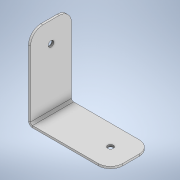
# Autodesk Inventor part: clamp
Saved by Autodesk Inventor 2021 (Build 250183000, 183)
## iProperties
Created: 2021-07-10
Part Number: clamp
Material: Generic
Document SubType Name: Sheet Metal
Designer: TARUN
Density: 1 g/cm^3
Sheet Metal Rule: Default_mm
Appearance: Default
Author: TARUN
Autodesk Inventor part; units mm, degrees
ref_plane "YZ Plane" through (0, 0, 0) normal (1, 0, 0) x (0, 1, 0)
ref_plane "XZ Plane" through (0, 0, 0) normal (0, 1, 0) x (-1, 0, 0)
ref_plane "XY Plane" through (0, 0, 0) normal (0, 0, 1) x (1, 0, 0)
sketch "Sketch1" plane through (0, 0, 0) normal (0, 1, 0) x (-1, 0, 0)
  line L0 (0, 5) -> (-20, 5)
  line L1 (-20, 5) -> (-20, -5)
  line L2 (-20, -5) -> (0, -5)
  line L3 (0, -5) -> (0, 5)
  point P0 (0, 0)
  dimension "d0" = 20
  dimension "d1" = 10
  measures "d0" distance of L0.start L0.end
  measures "d1" distance of L0.end L1.end
extrude "Plate1" add sketch "Sketch1" along normal blind 0.5
fillet "Corner Round1" radius 3 2 edges at (20, 0.25, 5) (20, 0.25, -5)
sketch "Sketch3" plane through (0, 0.5, 0) normal (0, 1, 0) x (1, 0, 0)
  line L0 (0, 5) -> (17, 5) projected
  line L1 (20, 2) -> (20, -2) projected
  point P0 (0, 0)
  point P1 (15, 0)
  point P2 (-17, 5)
  dimension "d22" = 5
  dimension "d23" = 5
  measures "d22" distance from line of L0 point (15, 0)
  measures "d23" distance from line of L1 point (15, 0)
hole "Hole2" at (15, 0.5, 0) direction (0, -1, 0) diameter 1.4 depth 0.5
sketch "Sketch4" plane through (0.5, 0, 5) normal (-1, 0, 0) x (0, -1, 0)
  line L0 (0, -10) -> (0, 0)
  line L1 (0, 0) -> (-20, 0)
  line L2 (-20, 0) -> (-20, -10)
  line L3 (-20, -10) -> (0, -10)
  constraints: 6 end point, 1 horizontal, 1 perpendicular, 1 vertical
edge flange "Flange1" height 20 angle 90 thickness 0.5 bend radius 0.5 thickness toward (-1, 0, 0) relief tear relief width 0.5 relief depth 0.25 edges at (0, 0.5, 0) wall of the first edge with corners at (0.5, 0, -5) (0.5, 0, 5) (0.5, 20, 5) (0.5, 20, -5)
bend "Bend1"
corner "Corner1"
fillet "Corner Round2" radius 3 2 edges at (0.25, 20, 5) (0.25, 20, -5)
sketch "Sketch5" plane through (0.5, 1, 5) normal (1, 0, 0) x (0, 0, -1)
  line L0 (7, 19) -> (3, 19) projected
  line L1 (0, 0) -> (0, 16) projected
  point P0 (5, -1)
  point P1 (5, 14)
  dimension "d42" = 5
  dimension "d43" = 5
  measures "d42" distance from line of L0 point (5, 14)
  measures "d43" distance from line of L1 point (5, 14)
hole "Hole3" at (0.5, 15, 0) direction (-1, 0, 0) diameter 1.4 depth 0.5
equation "\"d20\" = Thickness"
equation "\"d40\" = Thickness"
equation "\"d4\" = Thickness"
equation "\"d24\" = BendReliefWidth"
equation "\"d25\" = BendReliefDepth"
equation "\"d26\" = MinimumRemnant"
equation "\"d27\" = TransitionRadius"
equation "\"d30\" = BendRadius"
equation "\"d31\" = CornerReliefSize"
equation "\"d32\" = GapSize"
equation "\"d33\" = JacobiRadiusSize"
equation "\"BendRadius\" = Thickness"
equation "\"BendReliefWidth\" = Thickness"
equation "\"BendReliefDepth\" = 0.5 * Thickness"
equation "\"CornerReliefSize\" = 4 * Thickness"
equation "\"MinimumRemnant\" = 2 * Thickness"
equation "\"TransitionRadius\" = BendRadius"
equation "\"JacobiRadiusSize\" = BendRadius"
equation "\"GapSize\" = Thickness"
equation "\"Thickness\" = 0.5"
body "Solid1"
